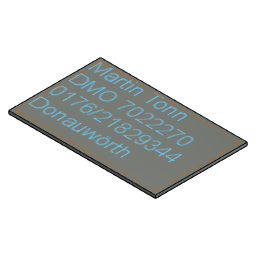
Schild (Autodesk Fusion 360 design; units mm, degrees)
Autodesk Fusion 360 part; units mm, degrees
sketch "Skizze1" plane through (0, 0, 0) normal (0, 1, 0) x (1, 0, 0)
  line L0 (0, 0) -> (40, 0)
  line L1 (40, 0) -> (40, 25)
  line L2 (40, 25) -> (0, 25)
  line L3 (0, 25) -> (0, 0)
  dimension "d1" = 40
  dimension "d2" = 25
  constraint horizontal L0
  constraint vertical L1
  constraint horizontal L2
  constraint vertical L3
  constraint coincident L0.start L3.end
  measures "d1" distance of L0.start L0.end
  measures "d2" distance of L0.start L2.end
extrude "Extrusion1" add sketch "Skizze1" along normal blind 0.8
sketch "Skizze2" plane through (0, 0.8, 0) normal (0, 1, 0) x (-1, 0, 0)
  line L0 (0, -25) -> (0, 0)
  line L1 (0, 0) -> (-40, 0)
  line L2 (-40, 0) -> (-40, -25)
  line L3 (-40, -25) -> (0, -25)
  line L4 (-0.9094, -1.0621) -> (-38.9956, -1.0184) construction
  line L5 (-38.9956, -1.0184) -> (-39.022, -23.9838) construction
  line L6 (-39.022, -23.9838) -> (-0.9358, -24.0275) construction
  line L7 (-0.9358, -24.0275) -> (-0.9094, -1.0621) construction
